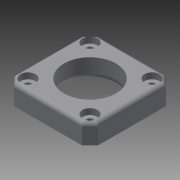
# Autodesk Inventor part: soporte02
Saved by Autodesk Inventor 2015 SP1 (Build 190203100, 203)
## iProperties
Created: 2015-06-16
Part Number: soporte02
Material: Generic
Document SubType Name: Modeling
Designer: pc
Density: 1 g/cm^3
Appearance: Default
Author: pc
Autodesk Inventor part; units mm, degrees
ref_plane "YZ Plane" through (0, 0, 0) normal (1, 0, 0) x (0, 1, 0)
ref_plane "XZ Plane" through (0, 0, 0) normal (0, 1, 0) x (-1, 0, 0)
ref_plane "XY Plane" through (0, 0, 0) normal (0, 0, 1) x (1, 0, 0)
sketch "Sketch1" plane through (0, 0, 0) normal (0, 0, 1) x (1, 0, 0)
  line L0 (-21, -21) -> (21, -21)
  line L1 (21, -21) -> (21, 21)
  line L2 (21, 21) -> (-21, 21)
  line L3 (-21, 21) -> (-21, -21)
  line L4 (-21, 0) -> (21, 0)
  line L5 (21, 0) -> (19, 0)
  line L6 (0, -21) -> (0, 21)
  point P0 (0, 0)
  point P1 (0, 0)
  dimension "d0" = 42
  dimension "d1" = 42
  constraints: 14 end point, 5 midpoint, 3 horizontal, 2 parallel, 1 coincident, 1 perpendicular
  measures "d0" distance of L2.end L1.end
  measures "d1" distance of L1.end L0.end
extrude "Extrusion1" add sketch "Sketch1" along normal blind 10
sketch "Sketch2" plane through (0, 0, 10) normal (0, 0, 1) x (1, 0, 0)
  circle A0 centre (0, 0) radius 13
  circle A1 centre (-15.5, 15.5) radius 1.75
  circle A2 centre (15.5, 15.5) radius 1.75
  circle A3 centre (15.5, -15.5) radius 1.75
  circle A4 centre (-15.5, -15.5) radius 1.75
  line L0 (21, 21) -> (-21, 21) projected
  line L1 (-21, 21) -> (-21, -21) projected
  line L2 (-21, -21) -> (21, -21) projected
  line L3 (21, -21) -> (21, 21) projected
  line L4 (0, -21) -> (0, 21)
  line L5 (-21, 0) -> (21, 0)
  dimension "d5" = 26
  dimension "d6" = 3.5
  dimension "d7" = 31
  dimension "d8" = 31
  constraints: 5 centre point, 4 end point, 4 midpoint, 3 equal radius, 2 horizontal alignment, 2 symmetric about line, 2 vertical alignment, 1 coincident
  measures "d5" diameter of A0
  measures "d6" diameter of A1
  measures "d7" distance of A2.centre A1.centre
  measures "d8" distance of A4.centre A1.centre
extrude "Extrusion2" cut sketch "Sketch2" against normal through all contours L5 L4 A0 | A0 L4 L5 | L4 L5 A0 | A0 L5 L4 | A1 | A2 | A3 | A4
chamfer "Chamfer1" distance 4 angle 45 4 edges at (-21, -21, 5) (21, -21, 5) (21, 21, 5) (-21, 21, 5)
sketch "Sketch3" plane through (0, 0, 10) normal (0, 0, 1) x (1, 0, 0)
  circle A0 centre (15.5, -15.5) radius 1.75 projected
  circle A1 centre (-15.5, -15.5) radius 1.75 projected
  circle A2 centre (0, 0) radius 13 projected
  circle A3 centre (-15.5, 15.5) radius 1.75 projected
  circle A4 centre (15.5, 15.5) radius 1.75 projected
  line L0 (-21, 17) -> (-17, 21) projected
  line L1 (-21, 17) -> (-21, -17) projected
  line L2 (-17, -21) -> (-21, -17) projected
  line L3 (-17, -21) -> (17, -21) projected
  line L4 (21, -17) -> (17, -21) projected
  line L5 (21, -17) -> (21, 17) projected
  line L6 (17, 21) -> (21, 17) projected
  line L7 (17, 21) -> (-17, 21) projected
  circle A5 centre (15.5, -15.5) radius 3.75
  circle A6 centre (-15.5, -15.5) radius 3.75
  circle A7 centre (-15.5, 15.5) radius 3.75
  circle A8 centre (15.5, 15.5) radius 3.75
  dimension "d14" = 2
  dimension "d17" = 2
  dimension "d18" = 2
  dimension "d19" = 2
  constraints: 4 centre point
  measures "d14" radial gap between concentric circles of A0 A5
  measures "d17" radial gap between concentric circles of A1 A6
  measures "d18" radial gap between concentric circles of A3 A7
  measures "d19" radial gap between concentric circles of A4 A8
extrude "Extrusion4" cut sketch "Sketch3" against normal blind 3 contours A5 | A6 | A7 | A8
fillet "Fillet1" radius 3 1 edges at (-13, 0, 0)
fillet "Fillet2" radius 2 8 edges at (0, -21, 10) (-19, -19, 10) (-21, 0, 10) (-19, 19, 10) (0, 21, 10) (19, 19, 10) (21, 0, 10) (19, -19, 10)
body "Solid1"
